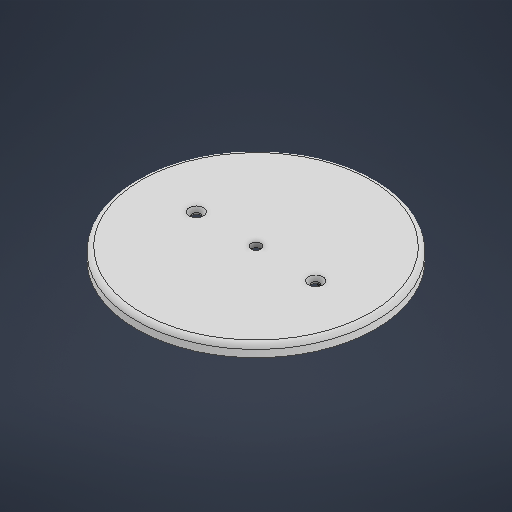
# Autodesk Inventor part: Spiegelhalterung
Saved by Autodesk Inventor 2025.2 (Build 292293000, 293)
## iProperties
Created: 2025-07-05
Part Number: Spiegelhalterung
Material: Generisch
Document SubType Name: Modeling
Designer: Faabs
Density: 1 g/cm^3
Appearance: Vorgabe
Author: Faabs
Autodesk Inventor part; units mm, degrees
ref_plane "YZ Plane" through (0, 0, 0) normal (1, 0, 0) x (0, 1, 0)
ref_plane "XZ Plane" through (0, 0, 0) normal (0, 1, 0) x (-1, 0, 0)
ref_plane "XY Plane" through (0, 0, 0) normal (0, 0, 1) x (1, 0, 0)
sketch "Skizze1" plane through (0, 0, 0) normal (0, 0, 1) x (1, 0, 0)
  circle A0 centre (0, 0) radius 50
  circle A1 centre (0, 0) radius 20
  circle A2 centre (0, 0) radius 2.05
  dimension "d0" = 100
  dimension "d1" = 40
  dimension "d2" = 4.1
  constraints: 3 centre point, 3 coincident
  measures "d0" diameter of A0
  measures "d1" diameter of A1
  measures "d2" diameter of A2
extrude "Extrusion1" add sketch "Skizze1" along normal blind 5 contours A0 | A1
extrude "Extrusion2" cut sketch "Skizze1" along normal blind 3 contours A1
sketch "Skizze3" plane through (0, 0, 0) normal (1, 0, 0) x (0, 1, 0)
  line L0 (0, 0) -> (20, 0)
  line L1 (20, 0) -> (20, -2)
  line L2 (20, -2) -> (24, -2)
  line L3 (24, -2) -> (24, 0)
  line L4 (50, 0) -> (-50, 0) projected
  line L5 (0, -3.4) -> (0, 6.4) projected
  dimension "d14" = 20
  dimension "d15" = 2
  dimension "d16" = 4
  constraints: 8 end point, 2 horizontal, 2 perpendicular, 1 point on line
  measures "d14" distance of L0.start L0.end
  measures "d15" distance of L0.end L1.end
  measures "d16" distance of L1.end L2.end
sketch "Skizze2" plane through (0, 0, 0) normal (0, 0, -1) x (-1, 0, 0)
  arc A0 (29.2471, -6.6791) -> (29.2471, 6.6791) centre (0, 0) ccw
  arc A1 (28.016, -7.4231) -> (29.2471, -6.6791) centre (28.2721, -6.4564) ccw
  line L0 (28.016, -7.4231) -> (21.1781, -5.6113)
  arc A2 (19.7185, -3.3437) -> (21.1781, -5.6113) centre (21.6904, -3.678) ccw
  arc A3 (19.7185, -3.3437) -> (19.7185, 3.3437) centre (0, 0) ccw
  arc A4 (21.1781, 5.6113) -> (19.7185, 3.3437) centre (21.6904, 3.678) ccw
  line L1 (21.1781, 5.6113) -> (28.016, 7.4231)
  arc A5 (29.2471, 6.6791) -> (28.016, 7.4231) centre (28.2721, 6.4564) ccw
  arc A6 (-29.2471, 6.6791) -> (-29.2471, -6.6791) centre (0, 0) ccw
  arc A7 (-28.016, 7.4231) -> (-29.2471, 6.6791) centre (-28.2721, 6.4564) ccw
  line L2 (-28.016, 7.4231) -> (-21.1781, 5.6113)
  arc A8 (-19.7185, 3.3437) -> (-21.1781, 5.6113) centre (-21.6904, 3.678) ccw
  arc A9 (-19.7185, 3.3437) -> (-19.7185, -3.3437) centre (0, 0) ccw
  arc A10 (-21.1781, -5.6113) -> (-19.7185, -3.3437) centre (-21.6904, -3.678) ccw
  line L3 (-21.1781, -5.6113) -> (-28.016, -7.4231)
  arc A11 (-29.2471, -6.6791) -> (-28.016, -7.4231) centre (-28.2721, -6.4564) ccw
  line L4 (21.1397, -5.7563) -> (27.9776, -7.5681)
  arc A12 (27.9776, -7.5681) -> (29.3933, -6.7125) centre (28.2721, -6.4564) ccw
  arc A13 (29.3933, -6.7125) -> (29.3933, 6.7125) centre (0, 0) ccw
  arc A14 (29.3933, 6.7125) -> (27.9776, 7.5681) centre (28.2721, 6.4564) ccw
  line L5 (27.9776, 7.5681) -> (21.1397, 5.7563)
  arc A15 (21.1397, 5.7563) -> (19.5706, 3.3186) centre (21.6904, 3.678) ccw
  arc A16 (19.5706, -3.3186) -> (19.5706, 3.3186) centre (0, 0) ccw
  arc A17 (19.5706, -3.3186) -> (21.1397, -5.7563) centre (21.6904, -3.678) ccw
  arc A18 (-19.5706, 3.3186) -> (-19.5706, -3.3186) centre (0, 0) ccw
  arc A19 (-19.5706, 3.3186) -> (-21.1397, 5.7563) centre (-21.6904, 3.678) ccw
  line L6 (-21.1397, 5.7563) -> (-27.9776, 7.5681)
  arc A20 (-27.9776, 7.5681) -> (-29.3933, 6.7125) centre (-28.2721, 6.4564) ccw
  arc A21 (-29.3933, 6.7125) -> (-29.3933, -6.7125) centre (0, 0) ccw
  arc A22 (-29.3933, -6.7125) -> (-27.9776, -7.5681) centre (-28.2721, -6.4564) ccw
  line L7 (-27.9776, -7.5681) -> (-21.1397, -5.7563)
  arc A23 (-21.1397, -5.7563) -> (-19.5706, -3.3186) centre (-21.6904, -3.678) ccw
  circle A24 centre (25, 0) radius 1.6
  circle A25 centre (-25, 0) radius 1.6
  dimension "d7" = 0.15
  dimension "d8" = 0.15
  dimension "d20" = 3.2
  dimension "d21" = 3.2
  constraints: 48 point on circle, 26 centre point, 16 end point, 14 other
  measures "d7" distance between parallel lines of L0 L4
  measures "d8" radial gap between concentric circles of A10 A23
  measures "d20" diameter of A24
  measures "d21" diameter of A25
revolve "Umdrehung1" add sketch "Skizze3" angle 360 about axis through (0, 0, -10) along (0, 0, 1)
extrude "Extrusion3" cut sketch "Skizze2" along normal mid plane 6 contours A1 L0 A2 A3 A4 L1 A5 A0 | A7 L2 A8 A9 A10 L3 A11 A6 | A17 A16 A15 L5 A14 A13 A12 L4 | A18 A23 L7 A22 A21 A20 L6 A19 | A24 | A25
extrude "Extrusion4" cut sketch "Skizze2" against normal blind 5 contours A24 | A25
fillet "Rundung1" radius 2 4 edges at (-19.5788, -4.0829, 0.5) (-19.5788, 4.0829, 0.5) (19.5788, -4.0829, 0.5) (19.5788, 4.0829, 0.5)
fillet "Rundung2" radius 2 2 edges at (0, 24, 0) (0, -24, 0)
fillet "Rundung3" radius 2 1 edges at (-50, 0, 5)
sketch "Skizze4" plane through (0, 0, 5) normal (0, 0, 1) x (1, 0, 0)
  circle A0 centre (-25, 0) radius 1.6 projected
  circle A1 centre (25, 0) radius 1.6 projected
  point P0 (0, 0)
  constraints: 2 coincident
hole "Bohrung1" at (-25, 0, 5) at (25, 0, 5) direction (0, 0, -1) diameter 3.2 depth 8 tip angle 118 countersink diameter 6 countersink angle 90
